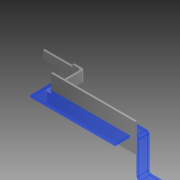
# Autodesk Inventor part: PosTerm
Saved by Autodesk Inventor 2014 (Build 180170000, 170)
## iProperties
Created: 2014-11-22
Part Number: PosTerm
Material: Nickel-Copper Alloy 400
Document SubType Name: Modeling
Designer: DV
Mass: 0.00760511 g
Surface Area: 0.191342 cm^2
Volume: 0.000861281 cm^3
Density: 8.83 g/cm^3
Appearance: Chrome - Polished
Author: DV
Autodesk Inventor part; units mm, degrees
ref_plane "YZ Plane" through (0, 0, 0) normal (1, 0, 0) x (0, 1, 0)
ref_plane "XZ Plane" through (0, 0, 0) normal (0, 1, 0) x (-1, 0, 0)
ref_plane "XY Plane" through (0, 0, 0) normal (0, 0, 1) x (1, 0, 0)
sketch "Sketch1" plane through (0, 0, 0) normal (0, 0, 1) x (1, 0, 0)
  circle A0 centre (3.019, 0) radius 2.2393 projected
  line L0 (3.8749, -0.95) -> (-0.5616, -0.95)
  line L1 (-0.5616, -0.2332) -> (-0.5616, 0.95)
  line L2 (-0.5616, 0.95) -> (3.8749, 0.95)
  line L3 (3.8749, 0.95) -> (3.8749, -0.95)
  line L4 (3.019, 0) -> (-3.8164, 0) construction
  line L5 (-0.5616, -0.95) -> (-2.881, -0.95)
  line L6 (-2.881, -0.95) -> (-2.881, -0.3679)
  line L7 (-2.881, -0.3679) -> (-1.3286, -0.3679)
  circle A1 centre (3.019, 0) radius 3.4 projected
  line L8 (-0.5616, -0.95) -> (-1.3286, -0.95)
  line L9 (-1.3286, -0.3679) -> (-1.3286, -0.2332)
  line L10 (-1.3286, -0.2332) -> (-0.5616, -0.2332)
  circle A2 centre (3.019, 0) radius 0.122
  point P0 (0, 0)
  dimension "d0" = 5.9
  dimension "d1" = 6.8
  dimension "d13" = 1.9
  dimension "d14" = 0.95
  constraints: 22 end point, 4 parallel, 4 perpendicular, 3 horizontal, 1 centre point, 1 coincident
  measures "d0" distance from line of L6 A1.centre
  measures "d1" diameter of A1
  measures "d13" distance between parallel lines of L0 L2
  measures "d14" distance from line of L2 L4.start
extrude "Extrusion1" add sketch "Sketch1" against normal blind 2 contours L2 L3 L0 A0 | A0 L0 A1 L2 | A1 L0 L5 L6 L7 L9 L10 L1 L2 picked at (2.6128, -0.6709) picked at (0.0739, 0.5857)
sketch "Sketch2" plane through (-2.881, -0.95, 0) normal (0, -1, 0) x (1, 0, 0)
  line L0 (6.7559, 0) -> (0, 0) projected
  line L1 (0, 0) -> (0, -2) projected
  line L2 (6.7559, -2) -> (0, -2) projected
  line L3 (6.7559, 0) -> (6.7559, -2) projected
  line L4 (0, -1.9) -> (1.873, -1.9)
  line L5 (2.227, -0.1) -> (6.7559, -0.1)
  line L6 (2.1, -1.873) -> (2.1, -0.227)
  line L7 (2, 0) -> (2, -1.773)
  arc A0 (1.873, -1.9) -> (2, -1.773) centre (1.873, -1.773) ccw
  arc A1 (2.227, -0.1) -> (2.1, -0.227) centre (2.227, -0.227) ccw
  line L8 (2.1, -1.9) -> (2.1, -2)
  line L9 (1.973, -2) -> (0, -2)
  line L10 (0, -2) -> (0, -1.9)
  line L11 (2.127, 0) -> (6.7559, 0)
  line L12 (6.7559, 0) -> (6.7559, -0.1)
  line L13 (2, -0.1) -> (2, -0.127)
  arc A2 (2.127, 0) -> (2, -0.127) centre (2.127, -0.127) ccw
  arc A3 (1.973, -2) -> (2.1, -1.873) centre (1.973, -1.873) ccw
  line L14 (6.7559, -0.1) -> (2.227, -0.1)
  line L15 (2.0029, -0.1) -> (2, -0.1)
  line L16 (0, -1.9) -> (1.873, -1.9)
  line L17 (2.0971, -1.9) -> (2.1, -1.9)
  point P0 (2.881, 0)
  point P1 (6.7559, -1.9)
  point P2 (0, -0.1)
  point P3 (2.1, 0)
  point P4 (2, -2)
  dimension "d4" = 0.1
  dimension "d5" = 0.1
  dimension "d6" = 2.1
  dimension "d7" = 0.1
  dimension "d8" = 0.127
  dimension "d9" = 0.127
  constraints: 28 end point, 16 point on line, 10 point on circle, 8 tangent, 7 perpendicular, 6 parallel, 4 centre point, 3 horizontal, 2 equal radius
  measures "d4" distance between parallel lines of L2 L4
  measures "d5" distance between parallel lines of L5 L0
  measures "d6" distance between parallel lines of L1 L6
  measures "d7" distance between parallel lines of L6 L7
  measures "d8" radius of A0
  measures "d9" radius of A2
extrude "Extrusion2" cut sketch "Sketch2" against normal blind 2 contours L3 L5 A1 L6 A3 L2 L1 L4 A0 L7 A2 L0 | A2 L15 L7 L0 keep common part
fillet "Fillet1" radius 0.127 1 edges at (-0.881, -0.5916, 0)
equation "\"d14\" = 0.5 * d13"
body "Solid1"
